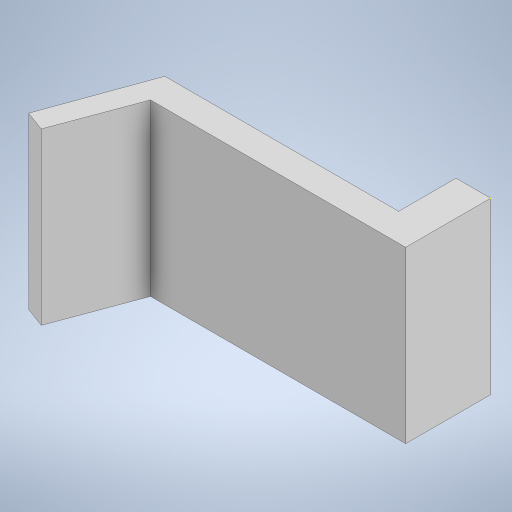
# Autodesk Inventor part: montageArm
Saved by Autodesk Inventor 2024 (Build 280153000, 153)
## iProperties
Created: 2024-11-21
Part Number: montageArm
Material: Generic
Document SubType Name: Modeling
Designer: domie
Density: 1 g/cm^3
Appearance: Default
Author: domie
Autodesk Inventor part; units mm, degrees
ref_plane "YZ Plane" through (0, 0, 0) normal (1, 0, 0) x (0, 1, 0)
ref_plane "XZ Plane" through (0, 0, 0) normal (0, 1, 0) x (-1, 0, 0)
ref_plane "XY Plane" through (0, 0, 0) normal (0, 0, 1) x (1, 0, 0)
sketch "Sketch1" plane through (0, 0, 0) normal (0, 1, 0) x (-1, 0, 0)
  line L0 (0, 0) -> (0, 20)
  line L1 (0, 20) -> (60, 20)
  line L2 (60, 20) -> (66.9645, 38.7482)
  line L3 (66.9645, 38.7482) -> (71.6515, 37.0071)
  line L4 (71.6515, 37.0071) -> (63.1538, 13.4957)
  line L5 (63.1538, 13.4957) -> (8.1538, 13.4957)
  line L6 (8.1538, 13.4957) -> (8.1538, 0)
  line L7 (8.1538, 0) -> (0, 0)
  dimension "d0" = 20
  dimension "d1" = 60
  dimension "d2" = 20
  dimension "d3" = 5
  dimension "d4" = 25
  dimension "d5" = 55
  constraints: 16 end point, 5 perpendicular, 1 vertical
  measures "d0" distance of L0.start L0.end
  measures "d1" distance of L0.end L1.end
  measures "d2" distance of L1.end L2.end
  measures "d3" distance of L2.end L3.end
  measures "d4" distance of L3.end L4.end
  measures "d5" distance of L4.end L5.end
extrude "Extrusion1" add sketch "Sketch1" along normal blind 40
sketch "Sketch2" plane through (0, 40, 0) normal (0, 1, 0) x (1, 0, 0)
  point P0 (0, 0)
body "Solid1"
